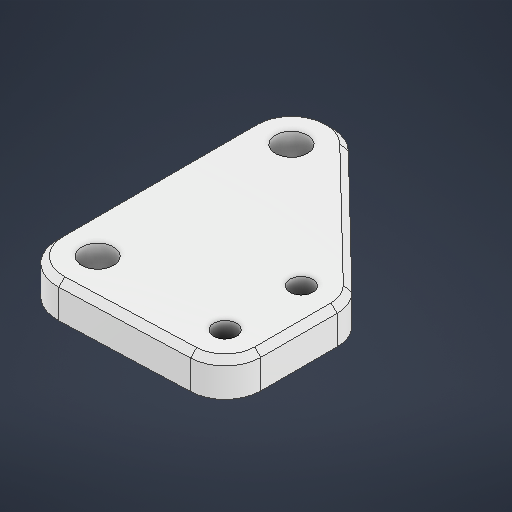
# Autodesk Inventor part: CNC-025-YAxisCableCarrierMount
Saved by Autodesk Inventor 2026.2 (Build 302298000, 298)
## iProperties
Created: 2026-06-25
Part Number: CNC-025-YAxisCableCarrierMount
Material: ABS Plastic
Document SubType Name: Modeling
Designer: Kenji
Density: 1.06 g/cm^3
Appearance: Smooth - White
Author: Kenji
Autodesk Inventor part; units mm, degrees
ref_plane "YZ Plane" through (0, 0, 0) normal (1, 0, 0) x (0, 1, 0)
ref_plane "XZ Plane" through (0, 0, 0) normal (0, 1, 0) x (-1, 0, 0)
ref_plane "XY Plane" through (0, 0, 0) normal (0, 0, 1) x (1, 0, 0)
sketch "Sketch1" plane through (0, 0, 0) normal (0, 1, 0) x (-1, 0, 0)
  circle A0 centre (0, 0) radius 2.1
  circle A1 centre (0, -25.4) radius 2.1
  circle A2 centre (-16.7115, 0) radius 1.5
  circle A3 centre (-16.7115, -10) radius 1.5
  circle A4 centre (0, 0) radius 5.275 construction
  circle A5 centre (0, -25.4) radius 5.275 construction
  circle A6 centre (-16.7115, 0) radius 4.675 construction
  circle A7 centre (-16.7115, -10) radius 4.675 construction
  line L0 (-0.1894, 5.2716) -> (-16.8793, 4.672)
  line L1 (5.275, 0) -> (5.275, -25.4)
  line L2 (-3.6758, -29.1834) -> (-19.9692, -13.353)
  line L3 (-21.3865, 0) -> (-21.3865, -10)
  arc A8 (-3.6758, -29.1834) -> (5.275, -25.4) centre (0, -25.4) ccw
  arc A9 (5.275, 0) -> (-0.1894, 5.2716) centre (0, 0) ccw
  arc A10 (-16.8793, 4.672) -> (-21.3865, 0) centre (-16.7115, 0) ccw
  arc A11 (-21.3865, -10) -> (-19.9692, -13.353) centre (-16.7115, -10) ccw
  dimension "d0" = 4.2
  dimension "d1" = 25.4
  dimension "d2" = 16.7115
  dimension "d3" = 3
  dimension "d4" = 10
  dimension "d5" = 3.175
  dimension "d6" = 3.175
  constraints: 16 point on circle, 12 centre point, 11 tangent, 8 end point, 7 equal radius, 2 coincident, 2 vertical alignment, 1 horizontal alignment, 1 vertical
  measures "d0" diameter of A0
  measures "d1" distance of A1.centre point (0, 0)
  measures "d2" distance of A2.centre point (0, 0)
  measures "d3" diameter of A2
  measures "d4" distance of A3.centre A2.centre
  measures "d5" radial gap between concentric circles of A0 A4
  measures "d6" radial gap between concentric circles of A6 A2
extrude "Extrusion1" add sketch "Sketch1" along normal blind 4.5994
chamfer "Chamfer1" distance 0.1984 angle 45 2 edges at (18.2115, 0, 0) (18.2115, 0, -10)
chamfer "Chamfer2" distance 0.7937 angle 45 8 edges at (-2.0537, 4.5994, -30.2588) (-5.275, 4.5994, -12.7) (-3.6624, 4.5994, 3.7964) (8.5344, 4.5994, 4.9718) (20.076, 4.5994, 3.2458) (21.3865, 4.5994, -5) (21.0176, 4.5994, -11.8201) (11.8225, 4.5994, -21.2682)
equation "\"d6\" = d5"
body "Solid1"
